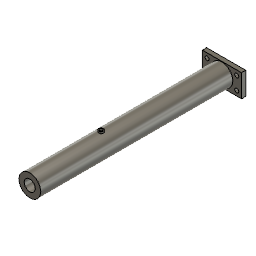
Measurement+Tube+Assembly (Autodesk Fusion 360 archive; units mm, degrees)
design "Measurement Tube"
Autodesk Fusion 360 part; units mm, degrees
(part 1 of 2)
sketch "Sketch1" plane through (0, 0, 0) normal (0, 0, 1) x (1, 0, 0)
  circle A0 centre (0, 0) radius 6.375
  circle A1 centre (0, 0) radius 12.5
  dimension "d1" = 25
  dimension "d2" = 12.75
  constraint coincident A0.centre A1.centre
  measures "d1" diameter of A1
  measures "d2" diameter of A0
extrude "Extrude1" add sketch "Sketch1" along normal blind 225 contours A0 | A1
extrude "Extrude19" cut sketch "Sketch1" along normal up to surface (225 mm away) contours A0
sketch "Sketch22" plane through (0, 0, 0) normal (0, 0, 1) x (1, 0, 0)
  line L0 (22.5, 13) -> (-22.5, 13)
  line L1 (-22.5, 13) -> (-22.5, -13)
  line L2 (-22.5, -13) -> (22.5, -13)
  line L3 (22.5, -13) -> (22.5, 13)
  circle A0 centre (0, 0) radius 6.375 construction
  circle A1 centre (0, 0) radius 12.5 construction
  line L4 (0, 0) -> (22.5, 0) construction
  line L5 (0, 0) -> (-22.5, 0) construction
  circle A2 centre (0, 0) radius 12.5
  circle A3 centre (17, 7.5) radius 2.25
  circle A4 centre (-17, 7.5) radius 2.25
  circle A5 centre (-17, -7.5) radius 2.25
  circle A6 centre (17, -7.5) radius 2.25
  point P0 (12.5, 0)
  point P1 (-12.5, 0)
  dimension "d150" = 10
  dimension "d151" = 10
  dimension "d152" = 13
  dimension "d155" = 4.5
  dimension "d156" = 17
  dimension "d157" = 17
  dimension "d158" = 17
  dimension "d159" = 17
  dimension "d160" = 4.5
  dimension "d161" = 4.5
  dimension "d162" = 4.5
  dimension "d163" = 7.5
  dimension "d164" = 7.5
  dimension "d165" = 7.5
  dimension "d166" = 7.5
  constraint horizontal L0
  constraint vertical L1
  constraint horizontal L2
  constraint vertical L3
  constraint coincident A0.centre A1.centre
  constraint midpoint L3 L4.end
  constraint horizontal L4
  constraint coincident A1 P0
  constraint coincident L4 P0
  constraint midpoint L1 L5.end
  constraint coincident A1 P1
  constraint coincident L5 P1
  constraint coincident P0 A2
  measures "d150" distance of L4.end P0
  measures "d151" distance of L5.end P1
  measures "d152" distance of L0 A0.centre
  measures "d155" diameter of A3
  measures "d156" horizontal distance of A0.centre A3.centre
  measures "d157" horizontal distance of A0.centre A4.centre
  measures "d158" horizontal distance of A0.centre A6.centre
  measures "d159" horizontal distance of A0.centre A5.centre
  measures "d160" diameter of A4
  measures "d161" diameter of A6
  measures "d162" diameter of A5
  measures "d163" distance of L4 A3.centre
  measures "d164" distance of L5 A4.centre
  measures "d165" distance of L4 A6.centre
  measures "d166" distance of L5 A5.centre
extrude "Mount Holes" add sketch "Sketch22" along normal blind 5
ref_plane "WorkPlane4" through (0, 6.4, 0) normal (0, 1, 0) x (0, 0, 1)
sketch "Sketch21" plane through (0, 6.4, 0) normal (0, 1, 0) x (1, 0, 0)
  circle A0 centre (0, -143.363) radius 1.7
  circle A1 centre (0, -143.363) radius 2.7
  line L0 (-12.5, -225) -> (12.5, -225)
  line L1 (22.5, 0) -> (-22.5, 0) construction
  line L2 (-22.5, 0) -> (-22.5, -5) construction
  line L3 (-22.5, -5) -> (22.5, -5) construction
  line L4 (22.5, -5) -> (22.5, 0) construction
  line L5 (0, -5) -> (0, -225) construction
  dimension "d137" = 3.4
  dimension "d138" = 5.4
  dimension "d167" = 81.637
  constraint concentric A0 A1
  constraint midpoint L3 L5.start
  constraint midpoint L0 L5.end
  constraint coincident A0.centre L5
  measures "d137" diameter of A0
  measures "d138" diameter of A1
  measures "d167" distance of A0.centre L0
extrude "Extrude17" add sketch "Sketch21" along normal blind 8
extrude "Extrude18" cut sketch "Sketch21" along normal blind 8 and the other way blind 2 contours A0
equation "d5 = 12.8 mm"
equation "d20 = 0.105 in"
equation "d22 = d20"
equation "d29 = 2.5 in"
equation "d129 = 7.5 mm"
equation "d136 = d5 / 2"
equation "d138 = d137 + 2 mm"
equation "d151 = d150"
equation "d157 = d156"
equation "d158 = d156"
equation "d159 = d156"
equation "d160 = d155"
equation "d161 = d155"
equation "d162 = d155"
equation "d164 = d163"
equation "d165 = d163"
equation "d166 = d163"
equation "d50 = d48 / 2"
equation "d51 = d50"
equation "d52 = d53"
equation "d53 = d46 / 2"
equation "d54 = 4.25 mm"
equation "d55 = d54"
equation "d56 = -d45"
equation "d58 = 4.5 mm"
equation "d59 = d58"
equation "d64 = d67"
equation "d67 = 154.736 mm"
equation "d70 = d67"
equation "d110 = d26 / 2"
equation "d111 = d16 / 2"
equation "d115 = -d29"
equation "d119 = -d29"
equation "d127 = 17 mm"
equation "d128 = d127"
equation "d130 = d129"
equation "d131 = 4.25 mm"
equation "d132 = d131"

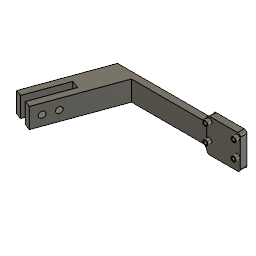
design "Camera Arm"
Autodesk Fusion 360 part; units mm, degrees
sketch "Sketch1" plane through (0, 0, 0) normal (0, 0, 1) x (1, 0, 0)
  circle A0 centre (10.5, -3.138) radius 1.2
  line L0 (-10.5, 12.5) -> (10.5, 12.5)
  arc A1 (-12.5, -10.5) -> (-10.5, -12.5) centre (-10.5, -10.5) ccw
  circle A2 centre (-10.5, -3.138) radius 1.2
  arc A3 (10.5, -12.5) -> (12.5, -10.5) centre (10.5, -10.5) ccw
  circle A4 centre (-10.5, 9.362) radius 1.2
  arc A5 (-10.5, 12.5) -> (-12.5, 10.5) centre (-10.5, 10.5) ccw
  line L1 (-12.5, -10.5) -> (-12.5, 10.5)
  line L2 (12.5, 10.5) -> (12.5, -10.5)
  arc A6 (12.5, 10.5) -> (10.5, 12.5) centre (10.5, 10.5) ccw
  circle A7 centre (10.5, 9.362) radius 1.2
  line L3 (10.5, -12.5) -> (-10.5, -12.5)
  point P0 (-12.5, 12.5)
  point P1 (12.5, 12.5)
  point P2 (-12.5, -12.5)
  dimension "d1" = 25
  dimension "d2" = 25
  dimension "d3" = 2.4
  dimension "d4" = 2
  dimension "d5" = 2
  dimension "d6" = 2
  dimension "d7" = 2
  dimension "d8" = 2
  dimension "d9" = 2
  dimension "d10" = 2
  dimension "d11" = 12.5
  dimension "d12" = 12.5
  dimension "d13" = 21.862
  dimension "d14" = 21.862
  dimension "d15" = 9.362
  dimension "d16" = 9.362
  dimension "d17" = 12.5
  dimension "d18" = 12.5
  constraint horizontal L0
  constraint vertical L2
  constraint horizontal L3
  constraint vertical L1
  constraint equal A2 A4
  constraint equal A0 A2
  constraint equal A0 A7
  constraint coincident P0 L0
  constraint coincident P0 L1
  constraint tangent L0 A5
  constraint tangent A5 L1
  constraint coincident P1 L0
  constraint coincident P1 L2
  constraint tangent L0 A6
  constraint tangent L2 A6
  constraint equal A5 A6
  constraint coincident P2 L3
  constraint coincident P2 L1
  constraint tangent A1 L3
  constraint tangent A1 L1
  constraint tangent A3 L2
  constraint tangent A3 L3
  measures "d1" distance of P0 P1
  measures "d2" distance of P0 P2
  measures "d3" diameter of A4
  measures "d4" distance of A7.centre L2
  measures "d5" distance of A0.centre L2
  measures "d6" distance of A2.centre L1
  measures "d7" distance of A4.centre L1
  measures "d8" radius of A5
  measures "d9" radius of A1
  measures "d10" radius of A3
  measures "d11" distance of origin L1
  measures "d12" distance of origin L0
  measures "d13" distance of A7.centre L3
  measures "d14" distance of A4.centre L3
  measures "d15" distance of A0.centre L3
  measures "d16" distance of A2.centre L3
  measures "d17" distance of origin L1
  measures "d18" distance of origin L0
extrude "Extrude1" add sketch "Sketch1" along normal blind 5
sketch "Sketch2" plane through (0, 0, 5) normal (0, 0, 1) x (1, 0, 0)
  circle A0 centre (-10.5, 9.362) radius 1.2
  circle A1 centre (10.5, -3.138) radius 1.2
  circle A2 centre (-10.5, -3.138) radius 1.2
  circle A3 centre (10.5, 9.362) radius 1.2
  arc A4 (12.5, 10.5) -> (10.5, 12.5) centre (10.5, 10.5) ccw
  line L0 (10.5, 12.5) -> (-10.5, 12.5)
  arc A5 (-10.5, 12.5) -> (-12.5, 10.5) centre (-10.5, 10.5) ccw
  line L1 (-12.5, 10.5) -> (-12.5, -10.5)
  arc A6 (-12.5, -10.5) -> (-10.5, -12.5) centre (-10.5, -10.5) ccw
  line L2 (-10.5, -12.5) -> (10.5, -12.5)
  arc A7 (10.5, -12.5) -> (12.5, -10.5) centre (10.5, -10.5) ccw
  line L3 (12.5, -10.5) -> (12.5, 10.5)
  circle A8 centre (-10.5, 9.362) radius 1.85
  circle A9 centre (10.5, 9.362) radius 1.85
  circle A10 centre (10.5, -3.138) radius 1.85
  circle A11 centre (-10.5, -3.138) radius 1.85
  dimension "d21" = 3.7
  dimension "d22" = 3.7
  dimension "d23" = 3.7
  dimension "d24" = 3.7
  constraint concentric A0 A8
  constraint concentric A3 A9
  constraint concentric A1 A10
  constraint concentric A2 A11
  measures "d21" diameter of A8
  measures "d22" diameter of A9
  measures "d23" diameter of A10
  measures "d24" diameter of A11
extrude "Extrude2" add sketch "Sketch2" along normal blind 3 contours A8 | A9 | A10 | A11
sketch "Sketch3" plane through (-12.5, 0, 0) normal (-1, 0, 0) x (0, 0, 1)
  line L0 (0, 10.5) -> (0, -10.5)
  line L1 (0, -10.5) -> (5, -10.5)
  line L2 (5, -10.5) -> (5, 10.5)
  line L3 (5, 10.5) -> (0, 10.5)
  line L4 (0, 7.5) -> (5, 7.5)
  line L5 (5, 7.5) -> (5, -7.5)
  line L6 (5, -7.5) -> (0, -7.5)
  line L7 (0, -7.5) -> (0, 7.5)
  dimension "d29" = 3
  dimension "d30" = 3
  constraint horizontal L4
  constraint vertical L5
  constraint horizontal L6
  constraint vertical L7
  constraint coincident L2 L5.end
  constraint coincident L0 L4.start
  measures "d29" distance of L3 L4
  measures "d30" distance of L1 L6
extrude "Extrude3" add sketch "Sketch3" along normal blind 68 contours L0 L2 L4 L5 L6 L7
fillet "Fillet1" radius 3 2 edges at (-12.5, 7.5, 2.5) (-12.5, -7.5, 2.5)
sketch "Sketch5" plane through (0, 7.5, 0) normal (0, 1, 0) x (-1, 0, 0)
  line L0 (15.5, 5) -> (15.5, 0)
  line L1 (15.5, 0) -> (80.5, 0)
  line L2 (80.5, 0) -> (80.5, 5)
  line L3 (80.5, 5) -> (15.5, 5)
  line L4 (80.5, 0) -> (94.2374, 0)
  line L5 (94.2374, 0) -> (80.5, 5)
  line L6 (84.001, 0) -> (85.1985, 3.2899)
  dimension "d38" = 20
  dimension "d39" = 5
  dimension "d40" = 5
  constraint coincident L1.end L2.start
  constraint perpendicular L2 L4
  constraint coincident L2.end L3.start
  constraint coincident L4 L6.start
  constraint coincident L5 L6.end
  constraint perpendicular L5 L6
  measures "d38" angle of L4 L5
  measures "d39" distance of L1.end L2.end
  measures "d40" distance of L2.end L6.end
extrude "Extrude5" add sketch "Sketch5" against normal up to surface (15 mm away) contours L2 L4 L5 L6
sketch "Sketch6" plane through (-11.0237, 0, 30.2873) normal (-0.34202, 0, 0.939693) x (0.939693, 0, 0.34202)
  line L0 (-78.9352, -7.5) -> (-73.9352, -7.5)
  line L1 (-73.9352, -7.5) -> (-73.9352, 7.5)
  line L2 (-73.9352, 7.5) -> (-78.9352, 7.5)
  line L3 (-78.9352, 7.5) -> (-78.9352, -7.5)
  line L4 (-78.9352, 7.5) -> (-73.9352, 7.5)
  line L5 (-73.9352, 7.5) -> (-73.9352, -7.5)
  line L6 (-73.9352, -7.5) -> (-78.9352, -7.5)
  line L7 (-78.9352, -7.5) -> (-78.9352, 7.5)
  constraint horizontal L4
  constraint vertical L5
  constraint horizontal L6
  constraint vertical L7
  constraint coincident L0.end L1.start
  constraint coincident L2.end L3.start
extrude "Extrude6" add sketch "Sketch6" along normal blind 55.398
sketch "Sketch7" plane through (-69.4763, 0, -25.2873) normal (0.939693, 0, 0.34202) x (0.34202, 0, -0.939693)
  line L0 (-32.2311, -7.5) -> (-32.2311, 7.5)
  line L1 (-32.2311, 7.5) -> (-87.6291, 7.5)
  line L2 (-87.6291, 7.5) -> (-87.6291, -7.5)
  line L3 (-87.6291, -7.5) -> (-32.2311, -7.5)
  line L4 (-87.6291, 0) -> (-32.2311, 0) construction
  circle A0 centre (-80.1291, 0) radius 2.25
  circle A1 centre (-70.1291, 0) radius 2.25
  dimension "d45" = 4.5
  dimension "d46" = 4.5
  dimension "d47" = 7.5
  dimension "d48" = 10
  constraint midpoint L2 L4.start
  constraint midpoint L0 L4.end
  constraint coincident L4 A0.centre
  constraint coincident L4 A1.centre
  measures "d45" diameter of A0
  measures "d46" diameter of A1
  measures "d47" distance of L2 A0.centre
  measures "d48" distance of A0.centre A1.centre
extrude "Extrude7" cut sketch "Sketch7" against normal up to surface (5 mm away) contours A0 | A1
sketch "Sketch8" plane through (0, 7.5, 0) normal (0, 1, 0) x (-1, 0, 0)
  line L0 (15.5, 5) -> (15.5, 0)
  line L1 (15.5, 0) -> (84.001, 0)
  line L2 (84.001, 0) -> (104.1457, 55.347)
  line L3 (104.1457, 55.347) -> (99.4472, 57.0571)
  line L4 (99.4472, 57.0571) -> (80.5, 5)
  line L5 (80.5, 5) -> (15.5, 5)
  line L6 (74.0085, 5) -> (93.7151, 59.1434)
  line L7 (93.7151, 59.1434) -> (89.0166, 60.8535)
  line L8 (89.0166, 60.8535) -> (68.6876, 5)
  line L9 (99.4472, 57.0571) -> (93.7151, 59.1434) construction
  dimension "d51" = 6.1
  dimension "d52" = 5
  constraint coincident L5 L6.start
  constraint perpendicular L6 L7
  constraint coincident L5 L8.end
  constraint parallel L4 L6
  constraint perpendicular L7 L8
  constraint coincident L3.end L4.start
  constraint perpendicular L4 L9
  measures "d51" distance of L4 L6
  measures "d52" distance of L6.end L7.end
extrude "Extrude8" add sketch "Sketch8" against normal up to surface (15 mm away) contours L5 L6 L7 L8
sketch "Sketch9" plane through (-59.0457, 0, -21.4909) normal (0.939693, 0, 0.34202) x (0.34202, 0, -0.939693)
  line L0 (-87.6291, -7.5) -> (-28.191, -7.5)
  line L1 (-28.191, -7.5) -> (-28.191, 7.5)
  line L2 (-28.191, 7.5) -> (-87.6291, 7.5)
  line L3 (-87.6291, 7.5) -> (-87.6291, -7.5)
  circle A0 centre (-80.1291, 0) radius 2.25
  circle A1 centre (-70.1291, 0) radius 2.25
extrude "Extrude9" cut sketch "Sketch9" against normal up to surface (5 mm away) contours A0 | A1
sketch "Sketch10" plane through (0, 7.5, 0) normal (0, 1, 0) x (-1, 0, 0)
  line L0 (15.5, 5) -> (15.5, 0)
  line L1 (15.5, 0) -> (84.001, 0)
  line L2 (84.001, 0) -> (104.1457, 55.347)
  line L3 (104.1457, 55.347) -> (99.4472, 57.0571)
  line L4 (99.4472, 57.0571) -> (80.5, 5)
  line L5 (80.5, 5) -> (74.0085, 5)
  line L6 (74.0085, 5) -> (93.7151, 59.1434)
  line L7 (93.7151, 59.1434) -> (89.0166, 60.8535)
  line L8 (89.0166, 60.8535) -> (68.6876, 5)
  line L9 (68.6876, 5) -> (15.5, 5)
  line L10 (89.0505, 28.4923) -> (83.3184, 30.5786)
  dimension "d57" = 30.398
  constraint coincident L4 L10.start
  constraint coincident L6 L10.end
  constraint perpendicular L6 L10
  measures "d57" distance of L3 L10
extrude "Extrude10" add sketch "Sketch10" against normal up to surface (15 mm away) contours L4 L5 L6 L10
equation "d17 = d11"
equation "d18 = d12"
equation "d22 = d21"
equation "d23 = d21"
equation "d24 = d21"
equation "d30 = d29"
equation "d40 = d39"
equation "d43 = 19.898 mm + 7.5 mm + 28 mm"
equation "d46 = d45"
equation "d57 = d43 - 25 mm"

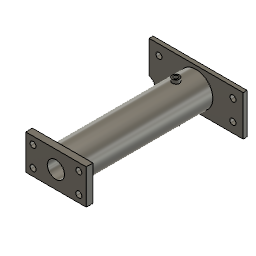
design "Measurement Tube Front Adapter"
Autodesk Fusion 360 part; units mm, degrees
sketch "Sketch1" plane through (0, 0, 0) normal (0, 0, 1) x (1, 0, 0)
  circle A0 centre (0, 0) radius 7
  circle A1 centre (0, 0) radius 12.5
  dimension "d1" = 25
  dimension "d2" = 14
  constraint coincident A0.centre A1.centre
  measures "d1" diameter of A1
  measures "d2" diameter of A0
extrude "Extrude1" add sketch "Sketch1" along normal blind 15 contours A0 | A1
sketch "Sketch2" plane through (0, 0, 15) normal (0, 0, 1) x (1, 0, 0)
  circle A0 centre (0, 0) radius 12.5
  circle A1 centre (0, 0) radius 6.375
  dimension "d5" = 12.75
  constraint concentric A0 A1
  measures "d5" diameter of A1
loft "Loft1" cut profiles "Sketch1", "Sketch2" section 1 contours A0 section 2 contours A1
extrude "Extrude2" add 1 faces at (10.4118, -0.621, 15) along direction (0, 0, 1) blind 92
sketch "Sketch17" plane through (0, 0, 107) normal (0, 0, 1) x (1, 0, 0)
  circle A0 centre (-17, -7.5) radius 2.25
  circle A1 centre (17, -7.5) radius 2.25
  circle A2 centre (0, 0) radius 6.375
  circle A3 centre (0, 0) radius 12.5
  line L0 (-22.5, 13) -> (22.5, 13)
  line L1 (22.5, 13) -> (22.5, -13)
  line L2 (22.5, -13) -> (-22.5, -13)
  line L3 (-22.5, -13) -> (-22.5, 13)
  line L4 (0, 0) -> (-22.5, 0) construction
  line L5 (0, 0) -> (22.5, 0) construction
  circle A4 centre (-17, 7.5) radius 2.25
  circle A5 centre (17, 7.5) radius 2.25
  point P0 (-12.5, 0)
  point P1 (12.5, 0)
  dimension "d112" = 4.5
  dimension "d113" = 4.5
  dimension "d147" = 10
  dimension "d148" = 10
  dimension "d149" = 7.5
  dimension "d150" = 13
  dimension "d151" = 17
  dimension "d152" = 17
  dimension "d153" = 7.5
  dimension "d154" = 17
  dimension "d155" = 7.5
  dimension "d156" = 4.5
  dimension "d157" = 4.5
  dimension "d158" = 17
  dimension "d159" = 7.5
  constraint horizontal L0
  constraint vertical L1
  constraint horizontal L2
  constraint vertical L3
  constraint coincident A2.centre A3.centre
  constraint midpoint L3 L4.end
  constraint midpoint L1 L5.end
  constraint horizontal L4
  constraint coincident A3 P0
  constraint coincident L4 P0
  constraint coincident L5 P1
  constraint coincident A3 P1
  measures "d112" diameter of A0
  measures "d113" diameter of A1
  measures "d147" distance of L4.end P0
  measures "d148" distance of L5.end P1
  measures "d149" distance of A0.centre L4
  measures "d150" distance of L2 L4
  measures "d151" horizontal distance of A0.centre A2.centre
  measures "d152" horizontal distance of A1.centre A2.centre
  measures "d153" distance of A1.centre L5
  measures "d154" horizontal distance of A2.centre A4.centre
  measures "d155" distance of L4 A4.centre
  measures "d156" diameter of A4
  measures "d157" diameter of A5
  measures "d158" horizontal distance of A2.centre A5.centre
  measures "d159" distance of L5 A5.centre
extrude "Extrude15" add sketch "Sketch17" against normal blind 5 contours A3 | L0 L1 L2 L3
sketch "Sketch18" plane through (0, 0, 0) normal (0, 0, -1) x (-1, 0, 0)
  circle A0 centre (-17, -7.5) radius 2.25
  circle A1 centre (17, -7.5) radius 2.25
  line L0 (-34.9564, 15) -> (34.9564, 15)
  line L1 (34.9564, 15) -> (34.9564, -15)
  line L2 (34.9564, -15) -> (-34.9564, -15)
  line L3 (-34.9564, -15) -> (-34.9564, 15)
  circle A2 centre (-27.4564, -7.5) radius 2.25
  circle A3 centre (0, 0) radius 7
  circle A4 centre (0, 0) radius 12.5
  line L4 (-22.5, -13) -> (22.5, -13)
  line L5 (22.5, -13) -> (22.5, 13)
  line L6 (22.5, 13) -> (-22.5, 13)
  line L7 (-22.5, 13) -> (-22.5, -13)
  circle A5 centre (0, 0) radius 12.5
  circle A6 centre (-17, 7.5) radius 2.25
  circle A7 centre (17, 7.5) radius 2.25
  circle A8 centre (-27.4564, 7.5) radius 2.25
  circle A9 centre (27.4564, 7.5) radius 2.25
  point P0 (0, -15)
  dimension "d122" = 4.5
  dimension "d124" = 7.5
  dimension "d125" = 7.5
  dimension "d160" = 34.9564
  dimension "d161" = 15
  dimension "d162" = 34.9564
  dimension "d163" = 15
  dimension "d164" = 7.5
  dimension "d165" = 7.5
  dimension "d166" = 4.5
  dimension "d167" = 7.5
  dimension "d168" = 7.5
  dimension "d169" = 4.5
  constraint horizontal L0
  constraint vertical L1
  constraint horizontal L2
  constraint vertical L3
  constraint midpoint L2 P0
  measures "d122" diameter of A2
  measures "d124" distance of L2 A2.centre
  measures "d125" distance of L3 A2.centre
  measures "d160" distance of A3.centre L3
  measures "d161" distance of A3.centre L2
  measures "d162" distance of L1.end P0
  measures "d163" distance of A3.centre L0
  measures "d164" distance of L0 A8.centre
  measures "d165" distance of L3 A8.centre
  measures "d166" diameter of A8
  measures "d167" distance of L1 A9.centre
  measures "d168" distance of L0 A9.centre
  measures "d169" diameter of A9
extrude "Extrude16" add sketch "Sketch18" against normal blind 3 contours A0 | A1 | L0 L1 L2 L3 | L4 L5 L6 L7 | A6 | A7
ref_plane "WorkPlane5" through (0, -7, 0) normal (0, 1, 0) x (0, 0, 1)
sketch "Sketch19" plane through (0, -7, 0) normal (0, 1, 0) x (1, 0, 0)
  line L0 (6.375, -15) -> (-6.375, -15)
  line L1 (0, -15) -> (0, -107) construction
  circle A0 centre (0, -18) radius 1.7
  circle A1 centre (0, -18) radius 2.7
  line L2 (6.375, -107) -> (-6.375, -107)
  dimension "d131" = 3.4
  dimension "d132" = 5.4
  dimension "d139" = 3
  constraint midpoint L0 L1.start
  constraint concentric A0 A1
  constraint coincident L1 A0.centre
  constraint midpoint L1.end L2
  measures "d131" diameter of A0
  measures "d132" diameter of A1
  measures "d139" distance of L0 A0.centre
extrude "Extrude17" add sketch "Sketch19" against normal blind 8
extrude "Extrude18" cut sketch "Sketch19" along normal blind 2 and the other way blind 8 contours A0
ref_plane "WorkPlane7" through (0, 7, 0) normal (0, 1, 0) x (0, 0, 1)
sketch "Sketch22" plane through (0, 7, 0) normal (0, 1, 0) x (1, 0, 0)
  circle A0 centre (0, -18) radius 1.7
  circle A1 centre (0, -18) radius 2.7
  point P0 (0, -18)
  dimension "d171" = 3.4
  dimension "d172" = 5.4
  constraint coincident P0 A0.centre
  measures "d171" diameter of A0
  measures "d172" diameter of A1
extrude "Extrude21" add sketch "Sketch22" along normal blind 8
extrude "Extrude22" cut sketch "Sketch22" along normal blind 8 and the other way blind 2 contours A0
sketch "Sketch23" plane through (0, 0, 0) normal (0, 0, -1) x (-1, 0, 0)
  line L0 (-34.9564, -15) -> (34.9564, -15)
  line L1 (34.9564, -15) -> (34.9564, 15)
  line L2 (34.9564, 15) -> (-34.9564, 15)
  line L3 (-34.9564, 15) -> (-34.9564, -15)
  circle A0 centre (-27.4564, 7.5) radius 2.25
  circle A1 centre (-27.4564, -7.5) radius 2.25
  circle A2 centre (27.4564, 7.5) radius 2.25
  circle A3 centre (0, 0) radius 7
  line L4 (34.9564, -15) -> (30.1724, -15)
  line L5 (34.9564, -9.125) -> (34.9564, -15)
  arc A4 (34.9564, -9.125) -> (30.1724, -15) centre (36.8966, -15.5902) ccw
  dimension "d181" = 4.784
  dimension "d182" = 5.875
  dimension "d183" = 6.75
  constraint horizontal L4
  constraint vertical L5
  constraint coincident L0.end L1.start
  measures "d181" distance of L0.end L4.end
  measures "d182" distance of L0.end L5.start
  measures "d183" radius of A4
extrude "Extrude23" cut sketch "Sketch23" against normal up to surface (3 mm away) contours L0 L1 L4 L5 A4
equation "d110 = 15 mm"
equation "d113 = d112"
equation "d116 = d110 / 2"
equation "d125 = d124"
equation "d130 = -d2 / 2"
equation "d132 = d131 + 2 mm"
equation "d148 = d147"
equation "d152 = d151"
equation "d153 = d149"
equation "d154 = d151"
equation "d155 = d149"
equation "d156 = d112"
equation "d157 = d112"
equation "d158 = d151"
equation "d159 = d149"
equation "d162 = d160"
equation "d163 = d161"
equation "d164 = d124"
equation "d165 = d124"
equation "d166 = d122"
equation "d167 = d124"
equation "d168 = d124"
equation "d169 = d122"
equation "d170 = ( d2 / 2 mm ) * 1 mm"
equation "d172 = d171 + 2 mm"
equation "d64 = d67"
equation "d67 = 40.00 mm"
equation "d70 = d67"
equation "d82 = -d67"
equation "d96 = d26 / 2"
equation "d97 = d16 / 2"
equation "d101 = -d29"
equation "d105 = -d29"
equation "d114 = 17 mm"
equation "d115 = d114"
equation "d117 = d116"
equation "d126 = d124"
equation "d127 = d124"

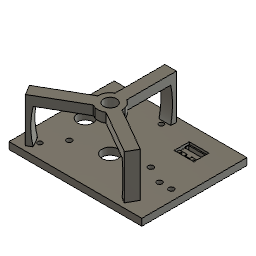
design "Strain Gauge Mount"
Autodesk Fusion 360 part; units mm, degrees
sketch "Sketch1" plane through (0, 0, 0) normal (0, 1, 0) x (1, 0, 0)
  line L0 (-47.5333, 52) -> (47.5333, 52) construction
  line L1 (47.5333, 52) -> (47.5333, -25) construction
  line L2 (47.5333, -25) -> (-47.5333, -25) construction
  line L3 (-47.5333, -25) -> (-47.5333, 52) construction
  line L4 (0, 8) -> (-6.9282, -4) construction
  line L5 (-6.9282, -4) -> (6.9282, -4) construction
  line L6 (6.9282, -4) -> (0, 8) construction
  line L7 (-2.5, 4.3301) -> (2.5, -4.3301) construction
  line L8 (2.5, -4.3301) -> (-42.5333, -30.3301) construction
  line L9 (-42.5333, -30.3301) -> (-47.5333, -21.6699) construction
  line L10 (-47.5333, -21.6699) -> (-2.5, 4.3301) construction
  line L11 (2.5, 4.3301) -> (-2.5, -4.3301) construction
  line L12 (-2.5, -4.3301) -> (42.5333, -30.3301) construction
  line L13 (42.5333, -30.3301) -> (47.5333, -21.6699) construction
  line L14 (2.5, 4.3301) -> (47.5333, -21.6699) construction
  line L15 (-5, 0) -> (-5, 52) construction
  line L16 (-5, 52) -> (5, 52) construction
  line L17 (5, 52) -> (5, 0) construction
  line L18 (5, 0) -> (-5, 0) construction
  line L19 (-5, 52) -> (-5, 2.8868)
  line L20 (-5, 2.8868) -> (-47.5333, -21.6699)
  line L21 (-47.5333, -21.6699) -> (-42.5333, -30.3301)
  line L22 (-42.5333, -30.3301) -> (0, -5.7735)
  line L23 (0, -5.7735) -> (42.5333, -30.3301)
  line L24 (42.5333, -30.3301) -> (47.5333, -21.6699)
  line L25 (47.5333, -21.6699) -> (5, 2.8868)
  line L26 (5, 2.8868) -> (5, 52)
  line L27 (5, 52) -> (-5, 52)
  circle A0 centre (0, 0) radius 10.5
  circle A1 centre (0, 0) radius 7
  dimension "d5" = 60
  dimension "d6" = 60
  dimension "d7" = 4
  dimension "d9" = 4
  dimension "d10" = 4
  dimension "d11" = 10
  dimension "d12" = 5
  dimension "d13" = 5
  dimension "d14" = 10
  dimension "d15" = 10
  dimension "d16" = 5
  dimension "d20" = 52
  dimension "d21" = 52
  dimension "d22" = 52
  dimension "d41" = 21
  dimension "d42" = 14
  constraint horizontal L0
  constraint vertical L1
  constraint horizontal L2
  constraint vertical L3
  constraint perpendicular L3 L5
  constraint parallel L6 L7
  constraint perpendicular L7 L8
  constraint coincident L3 L9.end
  constraint perpendicular L8 L9
  constraint perpendicular L7 L10
  constraint coincident A0.centre L7
  constraint perpendicular L11 L12
  constraint coincident L1 L13.end
  constraint perpendicular L12 L13
  constraint coincident A0.centre L11
  constraint perpendicular L13 L14
  constraint parallel L4 L11
  constraint coincident L0 L15.end
  constraint perpendicular L0 L15
  constraint coincident L0 L16.end
  constraint perpendicular L16 L17
  constraint perpendicular L17 L18
  constraint coincident A0.centre L18
  constraint coincident L15 L19.end
  constraint coincident L10 L19.end
  constraint perpendicular L9 L20
  constraint perpendicular L8 L21
  constraint coincident L12 L22.end
  constraint coincident L8 L22.end
  constraint coincident L17 L25.end
  constraint coincident L14 L25.end
  constraint coincident A0.centre A1.centre
  measures "d5" angle of L4 L5
  measures "d6" angle of L5 L6
  measures "d7" distance of A0.centre L5
  measures "d9" distance of A0.centre L6
  measures "d10" distance of A0.centre L4
  measures "d11" distance of L8.end L9.end
  measures "d12" distance of A0.centre L10
  measures "d13" distance of A0.centre L11.start
  measures "d14" distance of L12.end L13.end
  measures "d15" distance of L15 L17
  measures "d16" distance of A0.centre L15
  measures "d20" distance of L7.start L9.end
  measures "d21" distance of L11.start L13.end
  measures "d22" distance of L15.start L15.end
  measures "d41" diameter of A0
  measures "d42" diameter of A1
extrude "Extrude1" add sketch "Sketch1" along normal blind 6
sketch "Sketch2" plane through (0, 6, 0) normal (0, 1, 0) x (-1, 0, 0)
  line L0 (-5, -52) -> (5, -52)
  line L1 (5, -52) -> (5, -9.2331)
  line L2 (10.4961, 0.2864) -> (47.5333, 21.6699)
  line L3 (47.5333, 21.6699) -> (42.5333, 30.3301)
  line L4 (42.5333, 30.3301) -> (5.4961, 8.9467)
  line L5 (-5.4961, 8.9467) -> (-42.5333, 30.3301)
  line L6 (-42.5333, 30.3301) -> (-47.5333, 21.6699)
  line L7 (-47.5333, 21.6699) -> (-10.4961, 0.2864)
  line L8 (-5, -9.2331) -> (-5, -52)
  line L9 (5, -52) -> (-5, -52)
  line L10 (-5, -52) -> (-5, -47)
  line L11 (-5, -47) -> (5, -47)
  line L12 (5, -47) -> (5, -52)
  line L13 (43.2032, 19.1699) -> (38.2032, 27.8301)
  line L14 (43.2032, 19.1699) -> (47.5333, 21.6699)
  line L15 (47.5333, 21.6699) -> (42.5333, 30.3301)
  line L16 (42.5333, 30.3301) -> (38.2032, 27.8301)
  line L17 (-47.5333, 21.6699) -> (-42.5333, 30.3301)
  line L18 (-42.5333, 30.3301) -> (-38.2032, 27.8301)
  line L19 (-38.2032, 27.8301) -> (-43.2032, 19.1699)
  line L20 (-43.2032, 19.1699) -> (-47.5333, 21.6699)
  arc A0 (-10.4961, 0.2864) -> (-5, -9.2331) centre (0, 0) ccw
  arc A1 (5, -9.2331) -> (10.4961, 0.2864) centre (0, 0) ccw
  arc A2 (5.4961, 8.9467) -> (-5.4961, 8.9467) centre (0, 0) ccw
  dimension "d25" = 5
  dimension "d26" = 5
  dimension "d27" = 5
  constraint horizontal L9
  constraint vertical L10
  constraint horizontal L11
  constraint vertical L12
  constraint coincident L8 L10.end
  constraint coincident L0.end L1.start
  constraint coincident L2 L13.start
  constraint coincident L4 L13.end
  constraint perpendicular L4 L13
  constraint coincident L2.end L3.start
  constraint coincident L3.end L4.start
  constraint coincident L6.end L7.start
  constraint coincident L5.end L6.start
  constraint coincident L5 L18.end
  constraint coincident L7 L19.end
  constraint perpendicular L7 L19
  measures "d25" distance of L0.start L10.end
  measures "d26" distance of L13.start L2.end
  measures "d27" distance of L6.end L19.end
extrude "Extrude2" add sketch "Sketch2" along normal blind 30 contours L0 L1 L8 L9 L10 L11 L12 | L5 L6 L7 L17 L18 L19 L20 | L2 L3 L4 L13 L14 L15 L16
sketch "Sketch3" plane through (0, 36, 0) normal (0, 1, 0) x (-1, 0, 0)
  line L0 (43.2032, 19.1699) -> (47.5333, 21.6699)
  line L1 (47.5333, 21.6699) -> (42.5333, 30.3301)
  line L2 (42.5333, 30.3301) -> (38.2032, 27.8301)
  line L3 (38.2032, 27.8301) -> (43.2032, 19.1699)
  line L4 (-38.2032, 27.8301) -> (-43.2032, 19.1699)
  line L5 (-43.2032, 19.1699) -> (-10.4961, 0.2864)
  line L6 (-5, -9.2331) -> (-5, -47)
  line L7 (-5, -47) -> (5, -47)
  line L8 (5, -47) -> (5, -9.2331)
  line L9 (10.4961, 0.2864) -> (43.2032, 19.1699)
  line L10 (43.2032, 19.1699) -> (38.2032, 27.8301)
  line L11 (38.2032, 27.8301) -> (5.4961, 8.9467)
  line L12 (-5.4961, 8.9467) -> (-38.2032, 27.8301)
  line L13 (5, -47) -> (-5, -47)
  line L14 (-5, -47) -> (-5, -52)
  line L15 (-5, -52) -> (5, -52)
  line L16 (5, -52) -> (5, -47)
  line L17 (-43.2032, 19.1699) -> (-38.2032, 27.8301)
  line L18 (-38.2032, 27.8301) -> (-42.5333, 30.3301)
  line L19 (-42.5333, 30.3301) -> (-47.5333, 21.6699)
  line L20 (-47.5333, 21.6699) -> (-43.2032, 19.1699)
  line L21 (47.5333, 21.6699) -> (5, -9.2331)
  line L22 (5, -9.2331) -> (5, -52)
  line L23 (5, -52) -> (-5, -52)
  line L24 (-5, -52) -> (-10.4961, 0.2864)
  line L25 (-10.4961, 0.2864) -> (-47.5333, 21.6699)
  line L26 (-47.5333, 21.6699) -> (-42.5333, 30.3301)
  line L27 (-42.5333, 30.3301) -> (5.4961, 8.9467)
  line L28 (5.4961, 8.9467) -> (42.5333, 30.3301)
  line L29 (42.5333, 30.3301) -> (47.5333, 21.6699)
  line L30 (5, -9.5295) -> (-9.3062, -11.0333) construction
  line L31 (-10.7528, 0.4346) -> (-6.6754, 9.5928) construction
  line L32 (13.3677, -3.1535) -> (6.1603, 9.3301) construction
  circle A0 centre (0, 0) radius 10
  circle A1 centre (0, 0) radius 5.375
  arc A2 (-10.4961, 0.2864) -> (-5, -9.2331) centre (0, 0) ccw
  arc A3 (5, -9.2331) -> (10.4961, 0.2864) centre (0, 0) ccw
  arc A4 (5.4961, 8.9467) -> (-5.4961, 8.9467) centre (0, 0) ccw
  dimension "d33" = 10
  dimension "d34" = 10
  dimension "d35" = 10
  dimension "d40" = 10.75
  constraint coincident L0.end L1.start
  constraint coincident L8.end L21.end
  constraint coincident L15.end L16.start
  constraint coincident L14.end L15.start
  constraint coincident L5.end L24.end
  constraint coincident L19.end L20.start
  constraint coincident L18.end L19.start
  constraint coincident L11.end L27.end
  constraint coincident L1.end L2.start
  constraint coincident L8 L30.start
  constraint coincident L24 L30.end
  constraint perpendicular L24 L30
  constraint coincident L25 L31.start
  constraint perpendicular L27 L31
  constraint coincident L21 L32.start
  constraint coincident L11 L32.end
  constraint perpendicular L28 L32
  constraint concentric A0 A1
  measures "d33" distance of A0.centre L32
  measures "d34" distance of A0.centre L30
  measures "d35" distance of A0.centre L31
  measures "d40" diameter of A1
extrude "Extrude3" add sketch "Sketch3" along normal blind 8 contours L0 L1 L2 L3 L10 L28 L29 | L3 L4 L5 L6 L7 L8 L9 L10 L11 L12 L13 L17 L21 L22 L24 L25 L27 L28 A2 A3 A4 | L7 L13 L14 L15 L16 L22 L23 | L4 L17 L18 L19 L20 L25 L26 | A0 | A1
sketch "Sketch5" plane through (0, 44, 0) normal (0, 1, 0) x (-1, 0, 0)
  line L0 (40.8013, 29.3301) -> (5, 8.6603)
  arc A0 (5, 8.6603) -> (-5, 8.6603) centre (0, 0) ccw
  line L1 (-5, 8.6603) -> (-40.8013, 29.3301)
  line L2 (-40.8013, 29.3301) -> (-45.8013, 20.6699)
  line L3 (-45.8013, 20.6699) -> (-10, 0)
  arc A1 (-10, 0) -> (-5, -8.6603) centre (0, 0) ccw
  line L4 (-5, -8.6603) -> (-5, -50)
  line L5 (-5, -50) -> (5, -50)
  line L6 (5, -50) -> (5, -8.6603)
  arc A2 (5, -8.6603) -> (10, 0) centre (0, 0) ccw
  line L7 (10, 0) -> (45.8013, 20.6699)
  line L8 (45.8013, 20.6699) -> (40.8013, 29.3301)
  circle A3 centre (0, 0) radius 5.6417
  line L9 (-5.4961, 8.9467) -> (-42.5333, 30.3301)
  line L10 (-42.5333, 30.3301) -> (-47.5333, 21.6699)
  line L11 (-47.5333, 21.6699) -> (-10.4961, 0.2864)
  line L12 (-5, -9.2331) -> (-5, -52)
  line L13 (-5, -52) -> (5, -52)
  line L14 (5, -52) -> (5, -9.2331)
  line L15 (5, -9.2331) -> (7.2363, -7.6083)
  line L16 (47.5333, 21.6699) -> (42.5333, 30.3301)
  line L17 (42.5333, 30.3301) -> (5.4961, 8.9467)
  line L18 (-10.4961, 0.2864) -> (-10.2071, -2.4626)
  line L19 (5.4961, 8.9467) -> (2.9709, 10.0709)
  arc A4 (2.9709, 10.0709) -> (-5.4961, 8.9467) centre (0, 0) ccw
  arc A5 (-10.2071, -2.4626) -> (-5, -9.2331) centre (0, 0) ccw
  arc A6 (7.2363, -7.6083) -> (10.4961, 0.2864) centre (0, 0) ccw
  line L20 (10.4961, 0.2864) -> (47.5333, 21.6699)
  dimension "d39" = 11.2833
  constraint concentric A0 A3
  measures "d39" diameter of A3
loft "Loft1" cut profiles "Sketch5", "Sketch3" section 1 contours A3 section 2 contours A1
sketch "Sketch6" plane through (0, 6, 0) normal (0, 1, 0) x (-1, 0, 0)
  line L0 (-38.2032, 27.8301) -> (-43.2032, 19.1699)
  line L1 (-43.2032, 19.1699) -> (-10.4961, 0.2864)
  arc A0 (-10.4961, 0.2864) -> (-5, -9.2331) centre (0, 0) ccw
  line L2 (-5, -9.2331) -> (-5, -47)
  line L3 (-5, -47) -> (5, -47)
  line L4 (5, -47) -> (5, -9.2331)
  arc A1 (5, -9.2331) -> (10.4961, 0.2864) centre (0, 0) ccw
  line L5 (10.4961, 0.2864) -> (43.2032, 19.1699)
  line L6 (43.2032, 19.1699) -> (38.2032, 27.8301)
  line L7 (38.2032, 27.8301) -> (5.4961, 8.9467)
  arc A2 (5.4961, 8.9467) -> (-5.4961, 8.9467) centre (0, 0) ccw
  line L8 (-5.4961, 8.9467) -> (-38.2032, 27.8301)
  circle A3 centre (0, 0) radius 7
  dimension "d43" = 14
  constraint coincident A0.centre A1.centre
  measures "d43" diameter of A3
loft "Loft2" cut profiles "Sketch1", "Sketch6" section 1 contours L19 L20 L22 L23 L25 L26 A1 | L19 L20 A1 | L25 L26 A1 | L22 L23 A1 section 2 contours A3
sketch "Sketch9" plane through (2.5, 0, 4.3301) normal (0.5, 0, 0.866025) x (0.866025, 0, -0.5)
  line L0 (-9.2331, 6) -> (-47, 6)
  line L1 (-47, 6) -> (-47, 36)
  line L2 (-47, 36) -> (-9.2331, 36)
  line L3 (-9.2331, 36) -> (-9.2331, 44)
  line L4 (-9.2331, 44) -> (-52, 44)
  line L5 (-52, 44) -> (-52, 0)
  arc A0 (-47, 36) -> (-47, 6) centre (26.4847, 21) ccw
  line L6 (-47, 21) -> (81, 21) construction
  line L7 (-52, 0) -> (-9.2331, 0)
  line L8 (-9.2331, 0) -> (-9.2331, 6)
  dimension "d61" = 75
  constraint coincident L0.end L1.start
  constraint coincident L1.end L2.start
  constraint coincident L1 L6.start
  constraint perpendicular L1 L6
  constraint midpoint L1 L6.start
  measures "d61" radius of A0
extrude "Extrude7" cut sketch "Sketch9" against normal up to surface (10 mm away) contours L1 A0
sketch "Sketch10" plane through (-2.5, 0, 4.3301) normal (-0.5, 0, 0.866025) x (0.866025, 0, 0.5)
  line L0 (47, 6) -> (9.2331, 6)
  line L1 (52, 0) -> (52, 44)
  line L2 (52, 44) -> (9.2331, 44)
  line L3 (9.2331, 36) -> (47, 36)
  line L4 (47, 36) -> (47, 6)
  arc A0 (47, 6) -> (47, 36) centre (-26.4847, 21) ccw
  line L5 (9.2331, 0) -> (52, 0)
  line L6 (9.2331, 6) -> (9.2331, 0)
  line L7 (9.2331, 44) -> (9.2331, 36)
  dimension "d64" = 75
  constraint coincident L0.start L4.end
  constraint coincident L3.end L4.start
  measures "d64" radius of A0
extrude "Extrude8" cut sketch "Sketch10" against normal up to surface (10 mm away) contours L4 A0
sketch "Sketch11" plane through (5, 0, 0) normal (1, 0, 0) x (0, 0, -1)
  line L0 (47, 6) -> (9.2331, 6)
  line L1 (52, 0) -> (52, 44)
  line L2 (52, 44) -> (9.2331, 44)
  line L3 (47, 36) -> (47, 6)
  arc A0 (47, 6) -> (47, 36) centre (-26.4847, 21) ccw
  line L4 (9.2331, 36) -> (47, 36)
  line L5 (9.2331, 0) -> (52, 0)
  line L6 (9.2331, 6) -> (9.2331, 0)
  line L7 (9.2331, 44) -> (9.2331, 36)
  dimension "d67" = 75
  constraint coincident L0.start L3.end
  constraint coincident L3.start A0.end
  measures "d67" radius of A0
extrude "Extrude9" cut sketch "Sketch11" against normal up to surface (10 mm away) contours L3 A0
sketch "Sketch7" plane through (0, 6, 0) normal (0, 1, 0) x (-1, 0, 0)
  circle A0 centre (0, 0) radius 7
  line L0 (-43.2032, 19.1699) -> (-10.4961, 0.2864)
  arc A1 (-10.4961, 0.2864) -> (-5, -9.2331) centre (0, 0) ccw
  line L1 (-5, -9.2331) -> (-5, -47)
  line L2 (5, -47) -> (5, -9.2331)
  arc A2 (5, -9.2331) -> (10.4961, 0.2864) centre (0, 0) ccw
  line L3 (10.4961, 0.2864) -> (43.2032, 19.1699)
  line L4 (38.2032, 27.8301) -> (5.4961, 8.9467)
  arc A3 (5.4961, 8.9467) -> (-5.4961, 8.9467) centre (0, 0) ccw
  line L5 (-5.4961, 8.9467) -> (-38.2032, 27.8301)
  line L6 (52.5333, -56) -> (-61.5333, -56)
  line L7 (-61.5333, -56) -> (-61.5333, 34.3301)
  line L8 (-61.5333, 34.3301) -> (52.5333, 34.3301)
  line L9 (52.5333, 34.3301) -> (52.5333, -56)
  line L10 (47.5333, 21.6699) -> (42.5333, 30.3301)
  line L11 (-42.5333, 30.3301) -> (-47.5333, 21.6699)
  line L12 (-5, -52) -> (5, -52) construction
  line L13 (-38.2032, 27.8301) -> (-43.2032, 19.1699)
  line L14 (-5, -47) -> (5, -47)
  line L15 (43.2032, 19.1699) -> (38.2032, 27.8301)
  dimension "d51" = 4
  dimension "d139" = 5
  dimension "d141" = 14
  dimension "d142" = 4
  constraint horizontal L6
  constraint vertical L7
  constraint horizontal L8
  constraint vertical L9
  measures "d51" distance of L6 L12
  measures "d139" distance of L9 L10.start
  measures "d141" distance of L7 L11.end
  measures "d142" distance of L8 L10.end
extrude "Extrude5" add sketch "Sketch7" against normal blind 6 contours L6 L7 L8 L9
sketch "Sketch14" plane through (0, 0, 0) normal (0, -1, 0) x (1, 0, 0)
  line L0 (61.5333, 34.3301) -> (-52.5333, 34.3301)
  line L1 (-52.5333, 34.3301) -> (-52.5333, -56)
  line L2 (-52.5333, -56) -> (61.5333, -56)
  line L3 (61.5333, -56) -> (61.5333, 34.3301)
  circle A0 centre (27.456, -7.5) radius 2.25
  circle A1 centre (-27.456, 7.5) radius 2.25
  circle A2 centre (27.456, 7.5) radius 2.25
  line L4 (0, 0) -> (61.5333, 0) construction
  circle A3 centre (42.456, 0) radius 2.25
  circle A4 centre (52.456, 0) radius 2.25
  circle A5 centre (0, 0) radius 7
  dimension "d86" = 27.456
  dimension "d88" = 27.456
  dimension "d89" = 27.456
  dimension "d90" = 7.5
  dimension "d92" = 7.5
  dimension "d93" = 7.5
  dimension "d94" = 4.5
  dimension "d96" = 4.5
  dimension "d97" = 4.5
  dimension "d100" = 4.5
  dimension "d101" = 15
  dimension "d102" = 4.5
  dimension "d103" = 10
  dimension "d104" = 19.0773
  constraint coincident L3 L4.end
  constraint perpendicular L3 L4
  constraint coincident L4 A3.centre
  constraint coincident L4 A4.centre
  measures "d86" horizontal distance of L4.start A0.centre
  measures "d88" horizontal distance of L4.start A2.centre
  measures "d89" horizontal distance of L4.start A1.centre
  measures "d90" vertical distance of L4.start A0.centre
  measures "d92" vertical distance of L4.start A2.centre
  measures "d93" vertical distance of L4.start A1.centre
  measures "d94" diameter of A0
  measures "d96" diameter of A2
  measures "d97" diameter of A1
  measures "d100" diameter of A3
  measures "d101" horizontal distance of A0.centre A3.centre
  measures "d102" diameter of A4
  measures "d103" distance of A3.centre A4.centre
  measures "d104" distance of L3 A3.centre
extrude "Extrude12" cut sketch "Sketch14" against normal blind 8 contours A0 | A1 | A2 | A3 | A4
sketch "Sketch15" plane through (0, 6, 0) normal (0, 1, 0) x (-1, 0, 0)
  circle A0 centre (27.456, 7.5) radius 2.25
  circle A1 centre (-27.456, -7.5) radius 2.25
  circle A2 centre (-42.456, 0) radius 2.25
  circle A3 centre (-27.456, 7.5) radius 2.25
  circle A4 centre (-52.456, 0) radius 2.25
  line L0 (-5, -47) -> (5, -47)
  line L1 (5, -47) -> (5, -52)
  line L2 (5, -52) -> (-5, -52)
  line L3 (-5, -52) -> (-5, -47)
  line L4 (43.2032, 19.1699) -> (38.2032, 27.8301)
  line L5 (38.2032, 27.8301) -> (42.5333, 30.3301)
  line L6 (42.5333, 30.3301) -> (47.5333, 21.6699)
  line L7 (47.5333, 21.6699) -> (43.2032, 19.1699)
  line L8 (52.5333, 34.3301) -> (-61.5333, 34.3301)
  line L9 (-61.5333, 34.3301) -> (-61.5333, -56)
  line L10 (-61.5333, -56) -> (52.5333, -56)
  line L11 (52.5333, -56) -> (52.5333, 34.3301)
  circle A5 centre (0, 0) radius 7
  line L12 (-43.2032, 19.1699) -> (-47.5333, 21.6699)
  line L13 (-47.5333, 21.6699) -> (-42.5333, 30.3301)
  line L14 (-42.5333, 30.3301) -> (-38.2032, 27.8301)
  line L15 (-38.2032, 27.8301) -> (-43.2032, 19.1699)
  line L16 (-39.097, -32.667) -> (-25, -32.667) construction
  line L17 (-26.692, -32.667) -> (-26.692, -42.8778) construction
  circle A6 centre (-27.667, -32.667) radius 0.975
  line L18 (-27.667, -32.667) -> (-41.764, -32.667) construction
  line L19 (-25, -30) -> (-25, -42.8778)
  line L20 (-40.072, -32.667) -> (-40.072, -42.8778) construction
  line L21 (-41.764, -30) -> (-25, -30)
  circle A7 centre (-39.097, -32.667) radius 0.975
  line L22 (-41.764, -42.8778) -> (-41.764, -30)
  line L23 (-25, -42.8778) -> (-41.764, -42.8778)
  line L24 (-26.692, -39.1346) -> (-25, -39.1346) construction
  line L25 (-26.692, -39.1346) -> (-41.764, -39.1346) construction
  line L26 (-41.764, -39.1346) -> (-41.764, -34.6346)
  line L27 (-41.764, -34.6346) -> (-25, -34.6346)
  line L28 (-25, -34.6346) -> (-25, -39.1346)
  line L29 (-31.267, -34.6346) -> (-35.497, -34.6346)
  line L30 (-35.497, -34.6346) -> (-35.497, -32.6346)
  line L31 (-35.497, -32.6346) -> (-31.267, -32.6346)
  line L32 (-31.267, -32.6346) -> (-31.267, -34.6346)
  line L33 (-25.492, -41.8778) -> (-41.272, -41.8778)
  line L34 (-41.272, -41.8778) -> (-41.272, -39.1346)
  line L35 (-41.272, -39.1346) -> (-25.492, -39.1346)
  line L36 (-25.492, -39.1346) -> (-25.492, -41.8778)
  line L37 (-25.492, -39.1346) -> (-25, -39.1346)
  line L38 (-41.272, -39.1346) -> (-41.764, -39.1346)
  dimension "d105" = 12.8778
  dimension "d106" = 16.764
  dimension "d107" = 2.667
  dimension "d108" = 2.667
  dimension "d109" = 2.667
  dimension "d110" = 2.667
  dimension "d111" = 1.95
  dimension "d112" = 1.95
  dimension "d117" = 4.5
  dimension "d118" = 6.5
  dimension "d119" = 3.6
  dimension "d120" = 3.6
  dimension "d121" = 3.7432
  dimension "d122" = 1
  dimension "d123" = 1.2
  dimension "d124" = 1.2
  dimension "d143" = 30
  dimension "d144" = 25
  constraint coincident L16.start A7.centre
  constraint coincident L16.end L19
  constraint perpendicular L16 L19
  constraint coincident A6.centre L18.start
  constraint coincident L18.end L22
  constraint perpendicular L18 L22
  constraint coincident L20.start A7
  constraint coincident L20.start L18
  constraint coincident L20.end L23
  constraint tangent L20 A7
  constraint coincident L17.start L16
  constraint coincident L17.start A6
  constraint coincident L17.end L23
  constraint tangent L17 A6
  constraint coincident L24.start L17
  constraint perpendicular L19 L23
  constraint perpendicular L19 L21
  constraint perpendicular L21 L22
  constraint horizontal L23
  constraint coincident L19 L24.end
  constraint perpendicular L19 L24
  constraint coincident L22 L25.end
  constraint perpendicular L22 L25
  constraint vertical L26
  constraint horizontal L27
  constraint vertical L28
  constraint coincident L22 L26.end
  constraint horizontal L29
  constraint vertical L30
  constraint horizontal L31
  constraint vertical L32
  constraint coincident L27 L29.start
  constraint horizontal L33
  constraint vertical L34
  constraint horizontal L35
  constraint vertical L36
  constraint coincident L25 L34.end
  constraint perpendicular L22 L38
  measures "d105" distance of L22.start L21.start
  measures "d106" distance of L21.start L19.start
  measures "d107" distance of A6.centre L21
  measures "d108" distance of L16.start L21
  measures "d109" distance of L16.start L22
  measures "d110" distance of A6.centre L19
  measures "d111" diameter of A7
  measures "d112" diameter of A6
  measures "d117" distance of L25 L27
  measures "d118" distance of L25 L31
  measures "d119" distance of A6.centre L32
  measures "d120" distance of L16.start L30
  measures "d121" distance of L23 L25
  measures "d122" distance of L23 L33
  measures "d123" distance of L17 L36
  measures "d124" distance of L20 L34
  measures "d143" distance of A5.centre L21
  measures "d144" distance of A5.centre L19
extrude "Extrude13" cut sketch "Sketch15" against normal up to surface (6 mm away) contours A6 | L33 L34 L35 L36 | A7
extrude "Extrude14" cut sketch "Sketch15" against normal blind 2.7 contours L19 L22 L26 L27 L28 L29 L35 L37 L38 | L27 L29 L30 L31 L32
extrude "Extrude15" cut sketch "Sketch15" against normal blind 2 contours L19 L21 L22 L27 L30 L31 L32 | L19 L22 L23 L33 L34 L36 L37 L38
sketch "Sketch16" plane through (0, 6, 0) normal (0, 1, 0) x (-1, 0, 0)
  line L0 (-25, -30) -> (-25, -42.8778)
  line L1 (-25, -42.8778) -> (-41.764, -42.8778)
  line L2 (-41.764, -42.8778) -> (-41.764, -30)
  line L3 (-41.764, -30) -> (-25, -30)
  circle A0 centre (27.456, 7.5) radius 2.25
  circle A1 centre (-27.456, -7.5) radius 2.25
  circle A2 centre (-42.456, 0) radius 2.25
  circle A3 centre (-27.456, 7.5) radius 2.25
  circle A4 centre (-52.456, 0) radius 2.25
  line L4 (-5, -47) -> (5, -47)
  line L5 (5, -47) -> (5, -52)
  line L6 (5, -52) -> (-5, -52)
  line L7 (-5, -52) -> (-5, -47)
  line L8 (43.2032, 19.1699) -> (38.2032, 27.8301)
  line L9 (38.2032, 27.8301) -> (42.5333, 30.3301)
  line L10 (42.5333, 30.3301) -> (47.5333, 21.6699)
  line L11 (47.5333, 21.6699) -> (43.2032, 19.1699)
  line L12 (52.5333, 34.3301) -> (-61.5333, 34.3301)
  line L13 (-61.5333, 34.3301) -> (-61.5333, -56)
  line L14 (-61.5333, -56) -> (52.5333, -56)
  line L15 (52.5333, -56) -> (52.5333, 34.3301)
  circle A5 centre (0, 0) radius 7
  line L16 (-43.2032, 19.1699) -> (-47.5333, 21.6699)
  line L17 (-47.5333, 21.6699) -> (-42.5333, 30.3301)
  line L18 (-42.5333, 30.3301) -> (-38.2032, 27.8301)
  line L19 (-38.2032, 27.8301) -> (-43.2032, 19.1699)
  circle A6 centre (36.9738, -15.59) radius 6.75
  line L20 (36.9738, -15.59) -> (43.7238, -15.59) construction
  line L21 (36.9738, -15.59) -> (36.9738, -22.34) construction
  dimension "d132" = 13.5
  dimension "d145" = 36.9738
  dimension "d146" = 15.59
  dimension "d147" = 8.8095
  dimension "d148" = 33.66
  constraint coincident A6.centre L20.start
  constraint coincident A6 L20.end
  constraint horizontal L20
  constraint coincident A6 L21.end
  constraint perpendicular L20 L21
  measures "d132" diameter of A6
  measures "d145" horizontal distance of A5.centre A6.centre
  measures "d146" vertical distance of A5.centre A6.centre
  measures "d147" distance of L15 L20.end
  measures "d148" distance of L14 L21.end
extrude "Extrude16" cut sketch "Sketch16" against normal up to surface (6 mm away) contours A6
sketch "Sketch17" plane through (0, 6, 0) normal (0, 1, 0) x (-1, 0, 0)
  circle A0 centre (36.9738, -15.59) radius 6.75
  line L0 (-25, -30) -> (-25, -42.8778)
  line L1 (-25, -42.8778) -> (-41.764, -42.8778)
  line L2 (-41.764, -42.8778) -> (-41.764, -30)
  line L3 (-41.764, -30) -> (-25, -30)
  circle A1 centre (27.456, 7.5) radius 2.25
  circle A2 centre (-27.456, 7.5) radius 2.25
  circle A3 centre (-42.456, 0) radius 2.25
  circle A4 centre (-27.456, -7.5) radius 2.25
  circle A5 centre (-52.456, 0) radius 2.25
  line L4 (-5, -47) -> (5, -47)
  line L5 (5, -47) -> (5, -52)
  line L6 (5, -52) -> (-5, -52)
  line L7 (-5, -52) -> (-5, -47)
  line L8 (-43.2032, 19.1699) -> (-47.5333, 21.6699)
  line L9 (-47.5333, 21.6699) -> (-42.5333, 30.3301)
  line L10 (-42.5333, 30.3301) -> (-38.2032, 27.8301)
  line L11 (-38.2032, 27.8301) -> (-43.2032, 19.1699)
  line L12 (52.5333, 34.3301) -> (-61.5333, 34.3301)
  line L13 (-61.5333, 34.3301) -> (-61.5333, -56)
  line L14 (-61.5333, -56) -> (52.5333, -56)
  line L15 (52.5333, -56) -> (52.5333, 34.3301)
  circle A6 centre (0, 0) radius 7
  line L16 (38.2032, 27.8301) -> (42.5333, 30.3301)
  line L17 (42.5333, 30.3301) -> (47.5333, 21.6699)
  line L18 (47.5333, 21.6699) -> (43.2032, 19.1699)
  line L19 (43.2032, 19.1699) -> (38.2032, 27.8301)
  line L20 (-38.2032, 27.8301) -> (-43.2032, 19.1699)
  line L21 (43.2032, 19.1699) -> (38.2032, 27.8301)
  line L22 (-5, -47) -> (5, -47)
  line L23 (40.7032, 23.5) -> (0, 0) construction
  line L24 (0, 0) -> (-40.7032, 23.5) construction
  line L25 (0, 0) -> (0, -47) construction
  circle A7 centre (38.1051, 22) radius 2
  circle A8 centre (-38.1051, 22) radius 2
  circle A9 centre (0, -44) radius 2
  point P0 (39.8372, 23)
  point P1 (-39.8372, 23)
  point P2 (0, -46)
  dimension "d149" = 4
  dimension "d150" = 4
  dimension "d151" = 4
  dimension "d152" = 1
  dimension "d153" = 1
  dimension "d154" = 1
  constraint midpoint L19 L23.start
  constraint coincident A6.centre L23.end
  constraint midpoint L11 L24.end
  constraint midpoint L4 L25.end
  constraint coincident L23 A7.centre
  constraint coincident L24 A8.centre
  constraint coincident L25 A9.centre
  constraint coincident A7 P0
  constraint coincident L23 P0
  constraint coincident L24 P1
  constraint coincident A8 P1
  constraint coincident A9 P2
  constraint coincident L25 P2
  measures "d149" diameter of A7
  measures "d150" diameter of A9
  measures "d151" diameter of A8
  measures "d152" distance of L23.start P0
  measures "d153" distance of L25.end P2
  measures "d154" distance of L24.end P1
extrude "Extrude17" cut sketch "Sketch17" against normal up to surface (6 mm away) contours A7 | A8 | A9
equation "d6 = d5"
equation "d9 = d7"
equation "d10 = d7"
equation "d12 = d11 / 2"
equation "d13 = d14 / 2"
equation "d14 = d11"
equation "d15 = d11"
equation "d16 = d15 / 2"
equation "d21 = d20"
equation "d22 = d20"
equation "d23 = 6.00 mm"
equation "d26 = d25"
equation "d27 = d25"
equation "d34 = d33"
equation "d35 = d33"